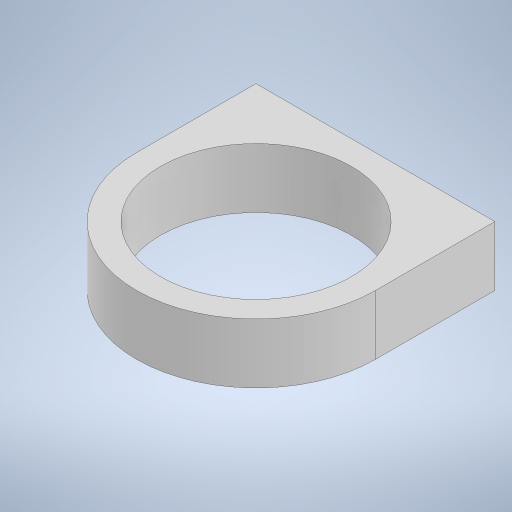
# Autodesk Inventor part: laterales
Saved by Autodesk Inventor 2024 (Build 280153000, 153)
## iProperties
Created: 2024-04-03
Part Number: laterales
Material: Generic
Document SubType Name: Modeling
Designer: compu
Density: 1 g/cm^3
Appearance: Default
Author: compu
Autodesk Inventor part; units mm, degrees
ref_plane "YZ Plane" through (0, 0, 0) normal (1, 0, 0) x (0, 1, 0)
ref_plane "XZ Plane" through (0, 0, 0) normal (0, 1, 0) x (-1, 0, 0)
ref_plane "XY Plane" through (0, 0, 0) normal (0, 0, 1) x (1, 0, 0)
sketch "Sketch1" plane through (0, 0, 0) normal (0, 1, 0) x (-1, 0, 0)
  line L0 (0, -19.6) -> (0, 19.6) projected
  line L1 (19.6, 0) -> (-19.6, 0) projected
  circle A0 centre (0, 0) radius 4
  circle A1 centre (0, 0) radius 11.2
  circle A2 centre (0, 0) radius 14
  line L2 (14, 0) -> (14, -14)
  line L3 (14, -14) -> (-14, -14)
  line L4 (-14, -14) -> (-14, 0)
  dimension "d0" = 8
  dimension "d1" = 22.4
  dimension "d2" = 28
  dimension "d3" = 28
  dimension "d4" = 14
  constraints: 6 end point, 3 centre point, 3 coincident, 2 perpendicular, 2 point on circle, 2 point on line, 1 tangent
  measures "d0" diameter of A0
  measures "d1" diameter of A1
  measures "d2" diameter of A2
  measures "d3" distance of L2.end L3.end
  measures "d4" distance from line of point (0, 0) L3
extrude "Extrusion1" add sketch "Sketch1" along normal blind 7 contours A2 L1 A1 L0 | L3 L4 A2 | L0 A1 L1 A2 | A2 L2 L3 | A2 L0 A1 L1 | L1 A1 L0 A2
body "Solid1"
